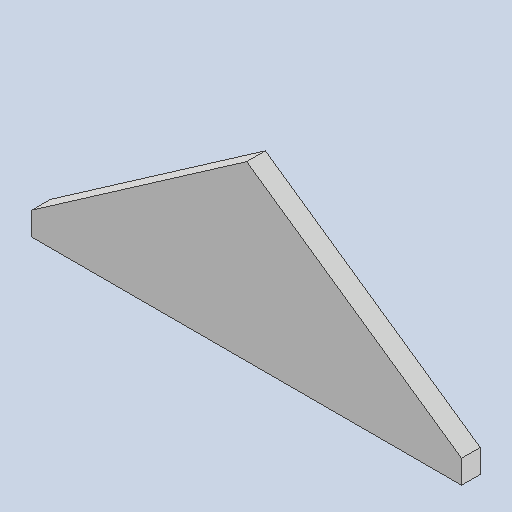
# Autodesk Inventor part: NDV-3003 Branch roof cap 01
Saved by Autodesk Inventor 2026.2 (Build 302298000, 298)
## iProperties
Created: 2026-10-05
Part Number: NDV-3003 Branch roof cap 01
Material: Generic
Document SubType Name: Sheet Metal
Designer: admin
Density: 1 g/cm^3
Sheet Metal Rule: Default_mm
Appearance: Default
Stock Number: Заглушка домика
Author: admin
Autodesk Inventor part; units mm, degrees
ref_plane "YZ Plane" through (0, 0, 0) normal (1, 0, 0) x (0, 1, 0)
ref_plane "XZ Plane" through (0, 0, 0) normal (0, 1, 0) x (-1, 0, 0)
ref_plane "XY Plane" through (0, 0, 0) normal (0, 0, 1) x (1, 0, 0)
derived "NDV-0010 Parameters 01.ipt"
sketch "sk_cap" plane through (0, 0, 0) normal (0, 0, 1) x (1, 0, 0)
  line L0 (-23, 0) -> (23, 0)
  line L1 (23, 0) -> (23, 2.5)
  line L2 (23, 2.5) -> (0, 18.5)
  line L3 (0, 18.5) -> (-23, 2.5)
  line L4 (-23, 2.5) -> (-23, 0)
  point P0 (0, 0)
  dimension "d1" = 46
  dimension "d2" = 2.5
  dimension "d3" = 18.5
  measures "d1" distance of L0.start L0.end
  measures "d2" distance of L0.end L1.end
  measures "d3" vertical distance of L0.start L2.end
extrude "Plate1" add sketch "sk_cap" along normal blind 2
equation "\"d1\" = Roof_cap_w"
equation "\"d2\" = Roof_cap_hs"
equation "\"d3\" = Roof_cap_h"
equation "\"d4\" = Thickness"
equation "\"Thickness\" = Roof_cap_t"
equation "\"BendRadius\" = Thickness"
equation "\"BendReliefWidth\" = Thickness"
equation "\"BendReliefDepth\" = 0.5 * Thickness"
equation "\"CornerReliefSize\" = 4 * Thickness"
equation "\"MinimumRemnant\" = 2 * Thickness"
equation "\"TransitionRadius\" = BendRadius"
equation "\"JacobiRadiusSize\" = BendRadius"
equation "\"GapSize\" = Thickness"
equation "\"Roof_cap_w\" = 46"
equation "\"Roof_cap_hs\" = 2.5"
equation "\"Roof_cap_h\" = 18.5"
equation "\"Roof_cap_t\" = 2"
body "Solid1"
